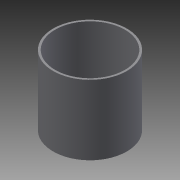
# Autodesk Inventor part: 091.061-FO1_BM_tube
Saved by Autodesk Inventor 2014 SP2 (Build 180246200, 246)
## iProperties
Created: 2020-02-04
Part Number: 091.061-FO1_BM_tube
Material: Generic
Catalog Web Link: www.cadenas.de
Description: FO1_basic_model_tube-Bimba FLAT-1
Vendor: BIMBA
Document SubType Name: Modeling
Designer: psadmin
Manufacturer: BIMBA
Mass: 1.78941 g
Surface Area: 48.2942 cm^2
Volume: 1.78941 cm^3
Density: 1 g/cm^3
Appearance: PSOLRGB-180-180-180
Category: PARTsolutions
Company: BIMBA
Title: 091.061-FO1_BM_tube
Author: Cadenas PARTsolutions
Comments: Bimba FLAT-1
PSOL_IDENT_0: {$CADENAS_DATA\23d-libs\bimba\bimba_brand\bimba_imperial\bimba_full_line\flat_cylinders\fo1\fo1_basi
PSOL_IDENT_1: c_model_tube.prj},207 {VTYP=3D},{NB=091.061-FO1_BM_tube},{LINA=091.061-FO1_BM_tube},{NN=FO1_basic_mo
PSOL_IDENT_2: del_tube},{DATE=22.01.2020 09:06:04},{GEOMDATE=17.09.2018 12:15:13},{VERSION=},{LINEID=30},{WBVAR=ST
PSOL_IDENT_3: ROKE,AB},{WBNUMERIC=STROKE}  {NB=091.061-FO1_BM_tube},{LINA=091.061-FO1_BM_tube},{KT=DUMMY},{PN=091.
PSOL_IDENT_4: 061-FO1_BM_tube},{BORE=1.06250000},{BOREPN=09},{STROKE=1.06100},{STROKEMIN=0.436},{AB=},{A=2.0000000
PSOL_IDENT_5: 0},{BA=0.88000},{BB=0.94000},{BC=1.5},{BD=2},{C=1.69000000},{DD=4.00000000},{D=0.13800000},{CPIL=0.1
PSOL_IDENT_6: 5600000},{DC=0.25000000},{DCP=0.14800000},{DCD=1.68700000},{ES=0.31250000},{EC=0.31250000},{ED=0.700
PSOL_IDENT_7: 00000},{F=0.50000000},{H=0.44000000},{J=0.50000000},{K=0.25000000},{L=0.40500000},{LDP=0.32300000},{
PSOL_IDENT_8: LP=0.12500000},{LPDP=0.59000000},{TD=1.11200000},{TDDP=0.21800},{TD1=1.10900},{TD2=1.12200},{TDIN=1.
PSOL_IDENT_9: 06200},{LSF=0.00000000},{LSFDP=0.00000000},{BC1=0.88000},{BC2=1.50000},{BC3=2.13000},{BC4=2.75000},{
PSOL_IDENT_10: BD1=1.38000},{BD2=2.00000},{BD3=2.63000},{BD4=3.25000},{TDAB=0.000},{TDA=1.122},{UNANG=7.500}
NN: FO1_basic_model_tube
NT: Bimba FLAT-1
NB: 091.061-FO1_BM_tube
NBSYN: $PN.
LINA: 091.061-FO1_BM_tube
PN: 091.061-FO1_BM_tube
BORE: 0
BOREPN: 09
STROKE: 1.061
AB: Standard
A: 2
BA: 0.88
BB: 0.94
C: 1.69
DD: 4
D: 0.138
CPIL: 0.156
DC: 0.25
DCP: 0.148
DCD: 1.687
ES: 0.3125
EC: 0.3125
ED: 0.7
F: 0.5
H: 0.44
J: 0.5
K: 0.25
L: 0.405
LDP: 0.323
LP: 0.125
LPDP: 0.59
TD: 1.112
TDDP: 0.218
TD1: 1.109
TD2: 1.122
TDIN: 1.062
LSF: 0
LSFDP: 0
BC1: 0.88
BC2: 1.5
BC3: 2.13
BC4: 2.75
BD1: 1.38
BD2: 2
BD3: 2.63
BD4: 3.25
TDAB: 0
UNANG: 7.5
SUPPLIER: BIMBA
ARTICLENO: 091.061-FO1_BM_tube
BOMINFO: 091.061-FO1_BM_tube
CREATOR: CADENAS GmbH
Autodesk Inventor part; units mm, degrees
ref_plane "YZ Plane" through (0, 0, 0) normal (1, 0, 0) x (0, 1, 0)
ref_plane "XZ Plane" through (0, 0, 0) normal (0, 1, 0) x (-1, 0, 0)
ref_plane "XY Plane" through (0, 0, 0) normal (0, 0, 1) x (1, 0, 0)
sketch "Sketch_4" plane through (0, 0, 0) normal (0, 0, 1) x (1, 0, 0)
  line L0 (0, 0) -> (0, 26.9494)
  line L1 (13.4874, 26.9494) -> (13.4874, 0)
  line L2 (13.4874, 0) -> (14.2494, 0)
  line L3 (14.2494, 0) -> (14.2494, 26.9494)
  line L4 (14.2494, 26.9494) -> (13.4874, 26.9494)
  constraints: 10 end point
revolve "Revolution1" add sketch "Sketch_4" angle 360 about axis through (0, 0, 0) along (0, -1, 0)
ref_plane "rod_to_part_XY" through (0, 13.4747, 0) normal (0, 1, 0) x (1, 0, 0)
ref_plane "rod_to_part_YZ" through (0, 13.4747, 0) normal (1, 0, 0) x (0, 0, -1)
ref_plane "rod_to_part_ZX" through (0, 13.4747, 0) normal (0, 0, -1) x (0, 1, 0)
ref_plane "to_road_XY" through (0, 13.4747, 0) normal (0, 1, 0) x (1, 0, 0)
ref_plane "to_road_YZ" through (0, 13.4747, 0) normal (1, 0, 0) x (0, 0, -1)
ref_plane "to_road_ZX" through (0, 13.4747, 0) normal (0, 0, -1) x (0, 1, 0)
ref_plane "track1_XY" through (-14.2494, 21.4122, 0) normal (0, 1, 0) x (1, 0, 0)
ref_plane "track1_YZ" through (-14.2494, 21.4122, 0) normal (1, 0, 0) x (0, 0, -1)
ref_plane "track1_ZX" through (-14.2494, 21.4122, 0) normal (0, 0, -1) x (0, 1, 0)
ref_plane "track1_u_XY" through (-14.2494, 5.5372, 0) normal (0, 1, 0) x (1, 0, 0)
ref_plane "track1_u_YZ" through (-14.2494, 5.5372, 0) normal (1, 0, 0) x (0, 0, -1)
ref_plane "track1_u_ZX" through (-14.2494, 5.5372, 0) normal (0, 0, -1) x (0, 1, 0)
ref_plane "track2_XY" through (0, 21.4122, -14.2494) normal (0, 1, 0) x (1, 0, 0)
ref_plane "track2_YZ" through (0, 21.4122, -14.2494) normal (1, 0, 0) x (0, 0, -1)
ref_plane "track2_ZX" through (0, 21.4122, -14.2494) normal (0, 0, -1) x (0, 1, 0)
ref_plane "track2_u_XY" through (0, 5.5372, -14.2494) normal (0, 1, 0) x (1, 0, 0)
ref_plane "track2_u_YZ" through (0, 5.5372, -14.2494) normal (1, 0, 0) x (0, 0, -1)
ref_plane "track2_u_ZX" through (0, 5.5372, -14.2494) normal (0, 0, -1) x (0, 1, 0)
ref_plane "track3_XY" through (14.2494, 21.4122, 0) normal (0, 1, 0) x (1, 0, 0)
ref_plane "track3_YZ" through (14.2494, 21.4122, 0) normal (1, 0, 0) x (0, 0, -1)
ref_plane "track3_ZX" through (14.2494, 21.4122, 0) normal (0, 0, -1) x (0, 1, 0)
ref_plane "track3_u_XY" through (14.2494, 5.5372, 0) normal (0, 1, 0) x (1, 0, 0)
ref_plane "track3_u_YZ" through (14.2494, 5.5372, 0) normal (1, 0, 0) x (0, 0, -1)
ref_plane "track3_u_ZX" through (14.2494, 5.5372, 0) normal (0, 0, -1) x (0, 1, 0)
ref_plane "track4_XY" through (0, 21.4122, 14.2494) normal (0, 1, 0) x (1, 0, 0)
ref_plane "track4_YZ" through (0, 21.4122, 14.2494) normal (1, 0, 0) x (0, 0, -1)
ref_plane "track4_ZX" through (0, 21.4122, 14.2494) normal (0, 0, -1) x (0, 1, 0)
ref_plane "track4_u_XY" through (0, 5.5372, 14.2494) normal (0, 1, 0) x (1, 0, 0)
ref_plane "track4_u_YZ" through (0, 5.5372, 14.2494) normal (1, 0, 0) x (0, 0, -1)
ref_plane "track4_u_ZX" through (0, 5.5372, 14.2494) normal (0, 0, -1) x (0, 1, 0)
ref_plane "tube_rear_XY" through (0, 26.9494, 0) normal (0, 1, 0) x (1, 0, 0)
ref_plane "tube_rear_YZ" through (0, 26.9494, 0) normal (1, 0, 0) x (0, 0, -1)
ref_plane "tube_rear_ZX" through (0, 26.9494, 0) normal (0, 0, -1) x (0, 1, 0)
ref_plane "tube_rod_guide_XY" through (0, 0, 0) normal (0, 1, 0) x (1, 0, 0)
ref_plane "tube_rod_guide_YZ" through (0, 0, 0) normal (1, 0, 0) x (0, 0, -1)
ref_plane "tube_rod_guide_ZX" through (0, 0, 0) normal (0, 0, -1) x (0, 1, 0)
body "Solid1"
